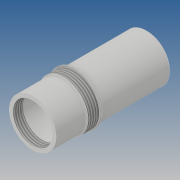
# Autodesk Inventor part: cartridge_locker_piston_cyl
Saved by Autodesk Inventor 2019 (Build 230136000, 136)
## iProperties
Created: 2019-03-17
Part Number: cartridge_locker_piston_cyl
Material: Générique
Document SubType Name: Modeling
Designer: Theo
Density: 1 g/cm^3
Appearance: Par défaut
Author: Theo
Autodesk Inventor part; units mm, degrees
ref_plane "YZ Plane" through (0, 0, 0) normal (1, 0, 0) x (0, 1, 0)
ref_plane "XZ Plane" through (0, 0, 0) normal (0, 1, 0) x (-1, 0, 0)
ref_plane "XY Plane" through (0, 0, 0) normal (0, 0, 1) x (1, 0, 0)
sketch "Esquisse3" plane through (0, 0, 0) normal (1, 0, 0) x (0, 1, 0)
  line L0 (0, 0) -> (0, -34.8052)
  line L1 (0, -45) -> (8, -45)
  line L2 (8, -45) -> (8, 0)
  line L3 (0, -45) -> (0, -46.5)
  line L4 (0, -46.5) -> (9.5, -46.5)
  line L5 (8, 0) -> (9.5, 0)
  line L6 (9.5, 0) -> (9.5, -12)
  line L7 (10, -12) -> (10, -17)
  line L8 (9.5, -19) -> (9.5, -46.5)
  line L9 (10, -17) -> (10.5, -17)
  line L10 (10.5, -17) -> (10.5, -17.5)
  line L11 (10.5, -17.5) -> (9.5, -19)
  line L12 (10, -12) -> (9.5, -12)
  dimension "d6" = 1.5
  dimension "d7" = 16
  dimension "d8" = 1.5
  dimension "d10" = 45
  dimension "d16" = 2
  dimension "d17" = 1.5
  dimension "d32" = 0.5
  dimension "d33" = 1.5
  dimension "d34" = 5
  dimension "d35" = 0.5
  dimension "d36" = 12
  constraints: 26 end point, 7 vertical, 5 horizontal, 1 horizontal alignment, 1 point on line
  measures "d6" distance between parallel lines of L4 L1
  measures "d7" diameter of L2 L0
  measures "d8" distance between parallel lines of L6 L2
  measures "d10" distance from line of L0.start L1
  measures "d16" distance between parallel lines of L7 L2
  measures "d17" distance between parallel lines of L8 L2
  measures "d32" distance of L7.end L9.end
  measures "d33" vertical distance of L10.end L8.start
  measures "d34" distance of L7.start L7.end
  measures "d35" distance of L9.end L10.end
  measures "d36" distance between parallel lines of L5 L12
revolve "Révolution1" add sketch "Esquisse3" angle 360 about axis through (0, 0, 0) along (0, 0, -1)
thread "Filetage2" size "M20x1" class "6g" standard "ISO Metric profile" full length
chamfer "Chanfrein4" distance 0.5 angle 45 3 edges at (0, -10, -12) (0, -9.5, -46.5) (0, -8, -45)
thread "Filetage3" size "M16x1" class "6H" standard "ISO Metric profile" length 4
equation "\"d6\" = d5"
equation "\"d35\" = d32"
equation "\"d5\" = 1.5"
